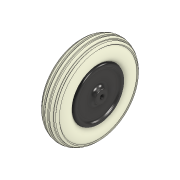
# Autodesk Inventor part: achterwiel
Saved by Autodesk Inventor 2020.3 (Build 243373000, 373)
## iProperties
Created: 2020-09-09
Part Number: achterwiel
Material: Stainless Steel
Document SubType Name: Modeling
Designer: Svend
Density: 8 g/cm^3
Appearance: Semi-Polished
Author: Svend
Autodesk Inventor part; units mm, degrees
ref_plane "YZ Plane" through (0, 0, 0) normal (1, 0, 0) x (0, 1, 0)
ref_plane "XZ Plane" through (0, 0, 0) normal (0, 1, 0) x (-1, 0, 0)
ref_plane "XY Plane" through (0, 0, 0) normal (0, 0, 1) x (1, 0, 0)
sketch "Sketch1" plane through (0, 0, 0) normal (0, 0, 1) x (1, 0, 0)
  circle A0 centre (0, 76) radius 24
  line L0 (-3, 97.5) -> (3, 97.5)
  line L1 (3, 97.5) -> (3, 102.5)
  line L2 (3, 102.5) -> (-3, 102.5)
  line L3 (-3, 102.5) -> (-3, 97.5)
  line L4 (-3, 97.5) -> (3, 102.5) construction
  line L5 (3, 97.5) -> (-3, 102.5) construction
  line L6 (-10.9993, 94.7154) -> (-5.4561, 97.0115)
  line L7 (-5.4561, 97.0115) -> (-7.3695, 101.6309)
  line L8 (-7.3695, 101.6309) -> (-12.9127, 99.3348)
  line L9 (-12.9127, 99.3348) -> (-10.9993, 94.7154)
  line L10 (-10.9993, 94.7154) -> (-7.3695, 101.6309) construction
  line L11 (-5.4561, 97.0115) -> (-12.9127, 99.3348) construction
  line L12 (-17.3241, 89.0815) -> (-13.0815, 93.3241)
  line L13 (-13.0815, 93.3241) -> (-16.617, 96.8597)
  line L14 (-16.617, 96.8597) -> (-20.8597, 92.617)
  line L15 (-20.8597, 92.617) -> (-17.3241, 89.0815)
  line L16 (-17.3241, 89.0815) -> (-16.617, 96.8597) construction
  line L17 (-13.0815, 93.3241) -> (-20.8597, 92.617) construction
  line L18 (-21.0115, 81.4561) -> (-18.7154, 86.9993)
  line L19 (-18.7154, 86.9993) -> (-23.3348, 88.9127)
  line L20 (-23.3348, 88.9127) -> (-25.6309, 83.3695)
  line L21 (-25.6309, 83.3695) -> (-21.0115, 81.4561)
  line L22 (-21.0115, 81.4561) -> (-23.3348, 88.9127) construction
  line L23 (-18.7154, 86.9993) -> (-25.6309, 83.3695) construction
  line L24 (-21.5, 73) -> (-21.5, 79)
  line L25 (-21.5, 79) -> (-26.5, 79)
  line L26 (-26.5, 79) -> (-26.5, 73)
  line L27 (-26.5, 73) -> (-21.5, 73)
  line L28 (-21.5, 73) -> (-26.5, 79) construction
  line L29 (-21.5, 79) -> (-26.5, 73) construction
  line L30 (-18.7154, 65.0007) -> (-21.0115, 70.5439)
  line L31 (-21.0115, 70.5439) -> (-25.6309, 68.6305)
  line L32 (-25.6309, 68.6305) -> (-23.3348, 63.0873)
  line L33 (-23.3348, 63.0873) -> (-18.7154, 65.0007)
  line L34 (-18.7154, 65.0007) -> (-25.6309, 68.6305) construction
  line L35 (-21.0115, 70.5439) -> (-23.3348, 63.0873) construction
  line L36 (-13.0815, 58.6759) -> (-17.3241, 62.9185)
  line L37 (-17.3241, 62.9185) -> (-20.8597, 59.383)
  line L38 (-20.8597, 59.383) -> (-16.617, 55.1403)
  line L39 (-16.617, 55.1403) -> (-13.0815, 58.6759)
  line L40 (-13.0815, 58.6759) -> (-20.8597, 59.383) construction
  line L41 (-17.3241, 62.9185) -> (-16.617, 55.1403) construction
  line L42 (-5.4561, 54.9885) -> (-10.9993, 57.2846)
  line L43 (-10.9993, 57.2846) -> (-12.9127, 52.6652)
  line L44 (-12.9127, 52.6652) -> (-7.3695, 50.3691)
  line L45 (-7.3695, 50.3691) -> (-5.4561, 54.9885)
  line L46 (-5.4561, 54.9885) -> (-12.9127, 52.6652) construction
  line L47 (-10.9993, 57.2846) -> (-7.3695, 50.3691) construction
  line L48 (3, 54.5) -> (-3, 54.5)
  line L49 (-3, 54.5) -> (-3, 49.5)
  line L50 (-3, 49.5) -> (3, 49.5)
  line L51 (3, 49.5) -> (3, 54.5)
  line L52 (3, 54.5) -> (-3, 49.5) construction
  line L53 (-3, 54.5) -> (3, 49.5) construction
  line L54 (10.9993, 57.2846) -> (5.4561, 54.9885)
  line L55 (5.4561, 54.9885) -> (7.3695, 50.3691)
  line L56 (7.3695, 50.3691) -> (12.9127, 52.6652)
  line L57 (12.9127, 52.6652) -> (10.9993, 57.2846)
  line L58 (10.9993, 57.2846) -> (7.3695, 50.3691) construction
  line L59 (5.4561, 54.9885) -> (12.9127, 52.6652) construction
  line L60 (17.3241, 62.9185) -> (13.0815, 58.6759)
  line L61 (13.0815, 58.6759) -> (16.617, 55.1403)
  line L62 (16.617, 55.1403) -> (20.8597, 59.383)
  line L63 (20.8597, 59.383) -> (17.3241, 62.9185)
  line L64 (17.3241, 62.9185) -> (16.617, 55.1403) construction
  line L65 (13.0815, 58.6759) -> (20.8597, 59.383) construction
  line L66 (21.0115, 70.5439) -> (18.7154, 65.0007)
  line L67 (18.7154, 65.0007) -> (23.3348, 63.0873)
  line L68 (23.3348, 63.0873) -> (25.6309, 68.6305)
  line L69 (25.6309, 68.6305) -> (21.0115, 70.5439)
  line L70 (21.0115, 70.5439) -> (23.3348, 63.0873) construction
  line L71 (18.7154, 65.0007) -> (25.6309, 68.6305) construction
  line L72 (21.5, 79) -> (21.5, 73)
  line L73 (21.5, 73) -> (26.5, 73)
  line L74 (26.5, 73) -> (26.5, 79)
  line L75 (26.5, 79) -> (21.5, 79)
  line L76 (21.5, 79) -> (26.5, 73) construction
  line L77 (21.5, 73) -> (26.5, 79) construction
  line L78 (18.7154, 86.9993) -> (21.0115, 81.4561)
  line L79 (21.0115, 81.4561) -> (25.6309, 83.3695)
  line L80 (25.6309, 83.3695) -> (23.3348, 88.9127)
  line L81 (23.3348, 88.9127) -> (18.7154, 86.9993)
  line L82 (18.7154, 86.9993) -> (25.6309, 83.3695) construction
  line L83 (21.0115, 81.4561) -> (23.3348, 88.9127) construction
  line L84 (13.0815, 93.3241) -> (17.3241, 89.0815)
  line L85 (17.3241, 89.0815) -> (20.8597, 92.617)
  line L86 (20.8597, 92.617) -> (16.617, 96.8597)
  line L87 (16.617, 96.8597) -> (13.0815, 93.3241)
  line L88 (13.0815, 93.3241) -> (20.8597, 92.617) construction
  line L89 (17.3241, 89.0815) -> (16.617, 96.8597) construction
  line L90 (5.4561, 97.0115) -> (10.9993, 94.7154)
  line L91 (10.9993, 94.7154) -> (12.9127, 99.3348)
  line L92 (12.9127, 99.3348) -> (7.3695, 101.6309)
  line L93 (7.3695, 101.6309) -> (5.4561, 97.0115)
  line L94 (5.4561, 97.0115) -> (12.9127, 99.3348) construction
  line L95 (10.9993, 94.7154) -> (7.3695, 101.6309) construction
  line L96 (-24, 76) -> (-24, 60)
  line L97 (24, 76) -> (24, 60)
  line L98 (-24, 60) -> (24, 60)
  line L99 (-37.1, 0) -> (37.1, 0) projected
  point P0 (0, 0)
  point P1 (0, 100)
  point P2 (-9.1844, 98.1731)
  point P3 (-16.9706, 92.9706)
  point P4 (-22.1731, 85.1844)
  point P5 (-22.1731, 66.8156)
  point P6 (-16.9706, 59.0294)
  point P7 (-9.1844, 53.8269)
  point P8 (0, 52)
  point P9 (9.1844, 53.8269)
  point P10 (16.9706, 59.0294)
  point P11 (22.1731, 66.8156)
  point P12 (22.1731, 85.1844)
  point P13 (16.9706, 92.9706)
  point P14 (9.1844, 98.1731)
  point P15 (-3, 99.8118)
  point P16 (-6.3407, 99.1472)
  point P17 (-11.884, 96.8511)
  point P18 (-14.7161, 94.9588)
  point P19 (-18.9588, 90.7161)
  point P20 (-17.8885, 60)
  point P21 (17.8885, 60)
  point P22 (23.8118, 73)
  point P23 (24, 73)
  point P24 (18.9588, 90.7161)
  point P25 (14.7161, 94.9588)
  point P26 (11.884, 96.8511)
  point P27 (6.3407, 99.1472)
  point P28 (3, 99.8118)
  dimension "d0" = 48
  dimension "d1" = 100
  dimension "d2" = 6
  dimension "d3" = 5
  dimension "d6" = 360
  dimension "d9" = 40
  constraints: 198 end point, 32 midpoint, 2 horizontal, 2 parallel, 2 vertical, 2 vertical alignment, 1 perpendicular, 180 other
  measures "d1" distance of point (0, 0) point (0, 100)
  measures "d2" distance of L2.end L1.end
  measures "d3" distance of L1.end L0.end
  measures "d9" distance from line of point (0, 100) L98
revolve "Revolution1" add sketch "Sketch1" angle 360 about axis through (-10, 0, 0) along (1, 0, 0) contours A0 L73 L72 L75 | L75 L72 L73 A0 L69 L66 L67 L63 L60 L98 L36 L37 L33 L30 L31 L27 L24 L25 L21 L18 L19 L15 L12 L13 L9 L6 L7 L3 L0 L1 L93 L90 L91 L87 L84 L85 L81 L78 L79 | L79 L78 L81 A0 | A0 L67 L66 L69 | L85 L84 L87 A0 | A0 L87 L86 L85 | A0 L98 L60 L63 | L91 L90 L93 A0 | A0 L93 L92 L91 | L98 A0 L37 L36 | L1 L0 L3 A0 | A0 L3 L2 L1 | L7 L6 L9 A0 | A0 L9 L8 L7 | A0 L31 L30 L33 | L13 L12 L15 A0 | A0 L15 L14 L13 | A0 L25 L24 L27 | L19 L18 L21 A0
sketch "Sketch2" plane through (0, 0, 0) normal (0, 1, 0) x (-1, 0, 0)
  line L0 (-17.8885, 60) -> (-17.8885, -60) projected
  line L1 (17.8885, 60) -> (17.8885, -60) projected
  circle A0 centre (-17.8885, 55) radius 5
  line L2 (-27.8885, 15) -> (-27.8885, -15)
  arc A1 (-27.8885, 15) -> (-17.8885, 25) centre (-27.8885, 25) ccw
  arc A2 (-17.8885, -25) -> (-27.8885, -15) centre (-27.8885, -25) ccw
  arc A3 (-17.8885, 45) -> (-20.8885, 51) centre (-25.3885, 45) ccw
  line L3 (-27.8885, 0) -> (20.8597, 0) construction
  line L4 (20.8597, 92.617) -> (20.8597, -92.617) construction
  line L5 (-17.8885, 60) -> (17.8885, 60) construction
  line L6 (0, 60) -> (0, -60) construction
  line L7 (3, 99.8118) -> (3, -99.8118) construction
  circle A4 centre (-17.8885, -55) radius 5
  arc A5 (-20.8885, -51) -> (-17.8885, -45) centre (-25.3885, -45) ccw
  circle A6 centre (17.8885, 55) radius 5
  line L8 (27.8885, 15) -> (27.8885, -15)
  arc A7 (17.8885, 25) -> (27.8885, 15) centre (27.8885, 25) ccw
  arc A8 (27.8885, -15) -> (17.8885, -25) centre (27.8885, -25) ccw
  arc A9 (20.8885, 51) -> (17.8885, 45) centre (25.3885, 45) ccw
  arc A10 (17.8885, -45) -> (20.8885, -51) centre (25.3885, -45) ccw
  circle A11 centre (17.8885, -55) radius 5
  line L9 (-24, 76) -> (-24, -76) projected
  line L10 (-12.8885, 0) -> (-27.8885, 0)
  line L11 (-17.8885, -60) -> (-12.8885, -60)
  line L12 (-12.8885, -60) -> (-12.8885, 60)
  line L13 (-12.8885, 60) -> (-17.8885, 60)
  line L14 (-17.8885, 60) -> (-17.8885, -60)
  point P0 (0, 0)
  point P1 (27.8885, 0)
  dimension "d11" = 10
  dimension "d12" = 30
  dimension "d13" = 10
  dimension "d14" = 10
  dimension "d15" = 5
  constraints: 26 symmetric about line, 24 point on circle, 18 end point, 12 centre point, 5 point on line, 4 midpoint, 4 tangent, 3 parallel, 2 perpendicular, 1 equal radius, 1 horizontal, 1 horizontal alignment, 1 line through centre, 1 vertical, 8 other
  measures "d11" diameter of A0
  measures "d12" distance of L2.start L2.end
  measures "d13" distance between parallel lines of L0 L2
  measures "d14" distance of A0.centre A3.start
  measures "d15" distance between parallel lines of L12 L14
revolve "Revolution2" add sketch "Sketch2" angle 360 about axis through (27.8885, 0, 0) along (-1, 0, 0) contours L10 L12 A4 L0 | L0 A2 L9 L10 | L9 A2 L2 L10 | L0 A4 A5 | L12 L11 A4 | A4 L0 | L0 A4
mirror "Mirror1" about plane through (0, 0, 0) normal (1, 0, 0) of "Revolution2"
sketch "Sketch3" plane through (27.8885, 0, 0) normal (1, 0, 0) x (0, 0, -1)
  circle A0 centre (0, 0) radius 15 projected
  circle A1 centre (0, 0) radius 15 projected
  circle A2 centre (0, 0) radius 5
  dimension "d17" = 10
  constraints: 1 centre point, 1 coincident
  measures "d17" diameter of A2
extrude "Extrusion1" cut sketch "Sketch3" against normal through all contours A2
fillet "Fillet1" radius 2 2 edges at (27.8885, 0, 15) (-27.8885, 0, 15)
body "Solid1"
